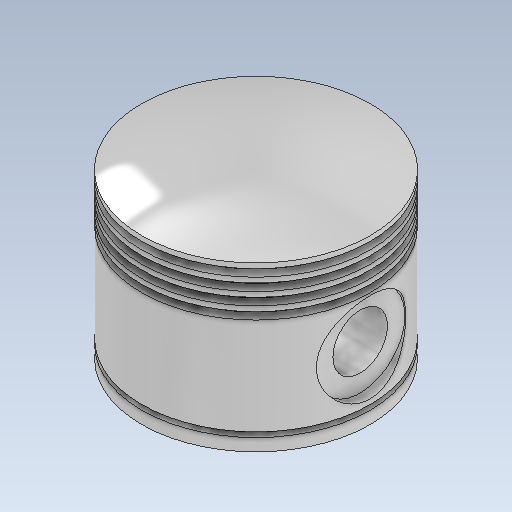
# Autodesk Inventor part: 15
Saved by Autodesk Inventor 2021 (Build 250183000, 183)
## iProperties
Category: 41
Created: 2021-07-27
Part Number: 15
Material: Alumínio 6061
Document SubType Name: Modeling
Designer: Giovanni
Density: 2.7 g/cm^3
Appearance: Alumínio - Polido
User Status: 1:2
Author: Giovanni
Keywords: 4
Autodesk Inventor part; units mm, degrees
ref_plane "XZ Plane" through (0, 0, 0) normal (0, 1, 0) x (-1, 0, 0)
sketch "Esboço1" plane through (0, 0, 0) normal (0, 0, 1) x (1, 0, 0)
  line L0 (0, 0) -> (0, 62)
  line L1 (37, 0) -> (37, 12)
  line L2 (37, 12) -> (38.5, 12)
  line L3 (38.5, 12) -> (38.5, 42)
  line L4 (38.5, 42) -> (37, 42)
  line L5 (37, 42) -> (37, 62)
  line L6 (37, 62) -> (0, 62)
  line L7 (0, 62) -> (0, 71.7)
  line L8 (37, 0) -> (46, 0)
  line L9 (46, 0) -> (46, 5)
  line L10 (46, 5) -> (42.5, 5)
  line L11 (42.5, 5) -> (42.5, 7)
  line L12 (42.5, 7) -> (46, 7)
  line L13 (46, 7) -> (46, 46)
  line L14 (46, 46) -> (42, 46)
  line L15 (42, 46) -> (42, 49)
  line L16 (42, 49) -> (46.0664, 49)
  line L17 (46.0664, 49) -> (46.0664, 51)
  line L18 (46.0664, 51) -> (42, 51)
  line L19 (42, 51) -> (42, 54)
  line L20 (42, 54) -> (46.0664, 54)
  line L21 (46.0664, 54) -> (46.0664, 56)
  line L22 (46.0664, 56) -> (42, 56)
  line L23 (42, 56) -> (42, 59)
  line L24 (42, 59) -> (46.0664, 59)
  line L25 (46.0664, 59) -> (46.0664, 61)
  line L26 (46.0664, 61) -> (42, 61)
  line L27 (42, 61) -> (42, 64)
  line L28 (42, 64) -> (46.0664, 64)
  line L29 (46.0664, 64) -> (46.0664, 66)
  arc A0 (46.0664, 66) -> (0, 71.7) centre (0, -117.3) ccw
  dimension "d0" = 62
  dimension "d1" = 74
  dimension "d2" = 77
  dimension "d3" = 12
  dimension "d4" = 30
  dimension "d5" = 9.7
  dimension "d6" = 85
  dimension "d7" = 92
  dimension "d8" = 5
  dimension "d9" = 2
  dimension "d10" = 46
  dimension "d11" = 4
  dimension "d12" = 3
  dimension "d15" = 2
  dimension "d20" = 189
  constraints: 60 end point, 16 point on line, 15 perpendicular, 3 vertical, 2 point on circle, 1 centre point, 1 horizontal alignment, 1 vertical alignment
  measures "d0" distance of L0.start L0.end
  measures "d1" diameter of L1 L0
  measures "d2" diameter of L3 L0
  measures "d3" distance of L1.start L1.end
  measures "d4" distance of L2.end L3.end
  measures "d5" distance of L0.end L7.end
  measures "d6" diameter of L10.end L0
  measures "d7" diameter of L8.end L0
  measures "d8" distance of L8.end L9.end
  measures "d9" distance of L9.end L12.end
  measures "d10" distance of L13.end L8.end
  measures "d11" distance of L13.end L14.end
  measures "d12" distance of L14.end L15.end
  measures "d15" distance of L20.end L21.end
  measures "d20" radius of A0
revolve "Revolução1" add sketch "Esboço1" angle 360 about axis through (0, 0, 0) along (0, -1, 0)
ref_plane "Plano de trabalho1" through (46, 26.5, 0) normal (1, 0, 0) x (0, 1, 0)
sketch "Esboço2" plane through (46, 26.5, 0) normal (1, 0, 0) x (0, 1, 0)
  circle A0 centre (0.5, 0) radius 18
  point P0 (-26.5, 0)
  dimension "d22" = 27
  dimension "d23" = 36
  constraints: 1 centre point, 1 horizontal alignment
  measures "d22" distance of point (-26.5, 0) A0.centre
  measures "d23" diameter of A0
extrude "Extrusão1" cut sketch "Esboço2" against normal blind 4
ref_plane "Plano de trabalho2" through (25, 0, 0) normal (1, 0, 0) x (0, 1, 0)
sketch "Esboço3" plane through (25, 0, 0) normal (1, 0, 0) x (0, 1, 0)
  circle A0 centre (27, 0) radius 19
  point P0 (0, 0)
  dimension "d27" = 27
  dimension "d28" = 38
  constraints: 1 centre point
  measures "d27" distance of A0.centre point (0, 0)
  measures "d28" diameter of A0
extrude "Extrusão2" add sketch "Esboço3" along normal up to next
sketch "Esboço4" plane through (42, 27, 0) normal (1, 0, 0) x (0, 0, -1)
  circle A0 centre (0, 0) radius 18 projected
  circle A1 centre (0, 0) radius 11
  point P0 (0, -27)
  dimension "d31" = 22
  constraints: 1 centre point, 1 coincident
  measures "d31" diameter of A1
extrude "Extrusão3" cut sketch "Esboço4" against normal blind 25 contours A1
mirror "Espelhamento1" about plane through (0, 0, 0) normal (1, 0, 0) of "Extrusão1", "Extrusão2", "Extrusão3"
